Autodesk Inventor part; units mm, degrees
(part 2 of 6)
  line L1007 (12.5, 39) -> (11.5, 39)
  line L1008 (11.5, 37.2) -> (11.5, 36.2)
  line L1009 (11.5, 36.2) -> (12.5, 36.2)
  line L1010 (12.5, 36.2) -> (12.5, 37.2)
  line L1011 (12.5, 37.2) -> (11.5, 37.2)
  line L1012 (4.542, 13.47) -> (5.542, 13.47)
  line L1013 (5.542, 13.47) -> (5.542, 14.47)
  line L1014 (5.542, 14.47) -> (4.542, 14.47)
  line L1015 (4.542, 14.47) -> (4.542, 13.47)
  line L1016 (6.142, 13.47) -> (7.142, 13.47)
  line L1017 (7.142, 13.47) -> (7.142, 14.47)
  line L1018 (7.142, 14.47) -> (6.142, 14.47)
  line L1019 (6.142, 14.47) -> (6.142, 13.47)
  line L1020 (7.142, 20.058) -> (6.142, 20.058)
  line L1021 (6.142, 20.058) -> (6.142, 19.058)
  line L1022 (6.142, 19.058) -> (7.142, 19.058)
  line L1023 (7.142, 19.058) -> (7.142, 20.058)
  line L1024 (5.542, 20.058) -> (4.542, 20.058)
  line L1025 (4.542, 20.058) -> (4.542, 19.058)
  line L1026 (4.542, 19.058) -> (5.542, 19.058)
  line L1027 (5.542, 19.058) -> (5.542, 20.058)
  line L1028 (28.0642, 20.3777) -> (28.7713, 19.6706)
  line L1029 (28.7713, 19.6706) -> (29.4784, 20.3777)
  line L1030 (29.4784, 20.3777) -> (28.7713, 21.0848)
  line L1031 (28.7713, 21.0848) -> (28.0642, 20.3777)
  line L1032 (29.1956, 19.2463) -> (29.9027, 18.5392)
  line L1033 (29.9027, 18.5392) -> (30.6098, 19.2463)
  line L1034 (30.6098, 19.2463) -> (29.9027, 19.9534)
  line L1035 (29.9027, 19.9534) -> (29.1956, 19.2463)
  line L1036 (20.985, 6.977) -> (19.985, 6.977)
  line L1037 (19.985, 6.977) -> (19.985, 5.977)
  line L1038 (19.985, 5.977) -> (20.985, 5.977)
  line L1039 (20.985, 5.977) -> (20.985, 6.977)
  line L1040 (19.385, 6.977) -> (18.385, 6.977)
  line L1041 (18.385, 6.977) -> (18.385, 5.977)
  line L1042 (18.385, 5.977) -> (19.385, 5.977)
  line L1043 (19.385, 5.977) -> (19.385, 6.977)
  line L1044 (17.981, 1.829) -> (18.981, 1.829)
  line L1045 (18.981, 1.829) -> (18.981, 2.829)
  line L1046 (18.981, 2.829) -> (17.981, 2.829)
  line L1047 (17.981, 2.829) -> (17.981, 1.829)
  line L1048 (19.881, 1.829) -> (20.881, 1.829)
  line L1049 (20.881, 1.829) -> (20.881, 2.829)
  line L1050 (20.881, 2.829) -> (19.881, 2.829)
  line L1051 (19.881, 2.829) -> (19.881, 1.829)
  line L1052 (18.931, 4.029) -> (19.931, 4.029)
  line L1053 (19.931, 4.029) -> (19.931, 5.029)
  line L1054 (19.931, 5.029) -> (18.931, 5.029)
  line L1055 (18.931, 5.029) -> (18.931, 4.029)
  circle A10 centre (7.874, 6.096) radius 0.5
  circle A11 centre (7.874, 43.053) radius 0.5
  circle A12 centre (27.94, 43.053) radius 0.5
  circle A13 centre (7.874, 6.096) radius 0.5
  circle A14 centre (7.874, 43.053) radius 0.5
  circle A15 centre (27.94, 43.053) radius 0.5
  circle A16 centre (3.302, 41.148) radius 2.667
  circle A17 centre (3.302, 41.148) radius 1.908
  circle A18 centre (3.302, 41.148) radius 1.908
  circle A19 centre (3.302, 41.148) radius 2.667
  circle A20 centre (32.258, 41.148) radius 2.667
  circle A21 centre (32.258, 41.148) radius 1.908
  circle A22 centre (32.258, 41.148) radius 1.908
  circle A23 centre (32.258, 41.148) radius 2.667
  line L1056 (33.0454, 18.9463) -> (33.0454, 19.6617)
  line L1057 (33.0454, 19.6617) -> (33.5513, 20.1676)
  line L1058 (33.5513, 20.1676) -> (34.2667, 20.1676)
  line L1059 (34.2667, 20.1676) -> (34.7726, 19.6617)
  line L1060 (34.7726, 19.6617) -> (34.7726, 18.9463)
  line L1061 (34.7726, 18.9463) -> (34.2667, 18.4404)
  line L1062 (34.2667, 18.4404) -> (33.5513, 18.4404)
  line L1063 (33.5513, 18.4404) -> (33.0454, 18.9463)
  circle A24 centre (33.909, 19.304) radius 0.8636
  circle A25 centre (33.909, 19.304) radius 0.8636
  line L1064 (33.0454, 18.9463) -> (33.0454, 19.6617)
  line L1065 (33.0454, 19.6617) -> (33.5513, 20.1676)
  line L1066 (33.5513, 20.1676) -> (34.2667, 20.1676)
  line L1067 (34.2667, 20.1676) -> (34.7726, 19.6617)
  line L1068 (34.7726, 19.6617) -> (34.7726, 18.9463)
  line L1069 (34.7726, 18.9463) -> (34.2667, 18.4404)
  line L1070 (34.2667, 18.4404) -> (33.5513, 18.4404)
  line L1071 (33.5513, 18.4404) -> (33.0454, 18.9463)
  line L1072 (33.0454, 16.4063) -> (33.0454, 17.1217)
  line L1073 (33.0454, 17.1217) -> (33.5513, 17.6276)
  line L1074 (33.5513, 17.6276) -> (34.2667, 17.6276)
  line L1075 (34.2667, 17.6276) -> (34.7726, 17.1217)
  line L1076 (34.7726, 17.1217) -> (34.7726, 16.4063)
  line L1077 (34.7726, 16.4063) -> (34.2667, 15.9004)
  line L1078 (34.2667, 15.9004) -> (33.5513, 15.9004)
  line L1079 (33.5513, 15.9004) -> (33.0454, 16.4063)
  circle A26 centre (33.909, 16.764) radius 0.8636
  circle A27 centre (33.909, 16.764) radius 0.8636
  line L1080 (33.0454, 16.4063) -> (33.0454, 17.1217)
  line L1081 (33.0454, 17.1217) -> (33.5513, 17.6276)
  line L1082 (33.5513, 17.6276) -> (34.2667, 17.6276)
  line L1083 (34.2667, 17.6276) -> (34.7726, 17.1217)
  line L1084 (34.7726, 17.1217) -> (34.7726, 16.4063)
  line L1085 (34.7726, 16.4063) -> (34.2667, 15.9004)
  line L1086 (34.2667, 15.9004) -> (33.5513, 15.9004)
  line L1087 (33.5513, 15.9004) -> (33.0454, 16.4063)
  line L1088 (33.0454, 13.8663) -> (33.0454, 14.5817)
  line L1089 (33.0454, 14.5817) -> (33.5513, 15.0876)
  line L1090 (33.5513, 15.0876) -> (34.2667, 15.0876)
  line L1091 (34.2667, 15.0876) -> (34.7726, 14.5817)
  line L1092 (34.7726, 14.5817) -> (34.7726, 13.8663)
  line L1093 (34.7726, 13.8663) -> (34.2667, 13.3604)
  line L1094 (34.2667, 13.3604) -> (33.5513, 13.3604)
  line L1095 (33.5513, 13.3604) -> (33.0454, 13.8663)
  circle A28 centre (33.909, 14.224) radius 0.8636
  circle A29 centre (33.909, 14.224) radius 0.8636
  line L1096 (33.0454, 13.8663) -> (33.0454, 14.5817)
  line L1097 (33.0454, 14.5817) -> (33.5513, 15.0876)
  line L1098 (33.5513, 15.0876) -> (34.2667, 15.0876)
  line L1099 (34.2667, 15.0876) -> (34.7726, 14.5817)
  line L1100 (34.7726, 14.5817) -> (34.7726, 13.8663)
  line L1101 (34.7726, 13.8663) -> (34.2667, 13.3604)
  line L1102 (34.2667, 13.3604) -> (33.5513, 13.3604)
  line L1103 (33.5513, 13.3604) -> (33.0454, 13.8663)
  line L1104 (33.0454, 11.3263) -> (33.0454, 12.0417)
  line L1105 (33.0454, 12.0417) -> (33.5513, 12.5476)
  line L1106 (33.5513, 12.5476) -> (34.2667, 12.5476)
  line L1107 (34.2667, 12.5476) -> (34.7726, 12.0417)
  line L1108 (34.7726, 12.0417) -> (34.7726, 11.3263)
  line L1109 (34.7726, 11.3263) -> (34.2667, 10.8204)
  line L1110 (34.2667, 10.8204) -> (33.5513, 10.8204)
  line L1111 (33.5513, 10.8204) -> (33.0454, 11.3263)
  circle A30 centre (33.909, 11.684) radius 0.8636
  circle A31 centre (33.909, 11.684) radius 0.8636
  line L1112 (33.0454, 11.3263) -> (33.0454, 12.0417)
  line L1113 (33.0454, 12.0417) -> (33.5513, 12.5476)
  line L1114 (33.5513, 12.5476) -> (34.2667, 12.5476)
  line L1115 (34.2667, 12.5476) -> (34.7726, 12.0417)
  line L1116 (34.7726, 12.0417) -> (34.7726, 11.3263)
  line L1117 (34.7726, 11.3263) -> (34.2667, 10.8204)
  line L1118 (34.2667, 10.8204) -> (33.5513, 10.8204)
  line L1119 (33.5513, 10.8204) -> (33.0454, 11.3263)
  line L1120 (33.0454, 8.7863) -> (33.0454, 9.5017)
  line L1121 (33.0454, 9.5017) -> (33.5513, 10.0076)
  line L1122 (33.5513, 10.0076) -> (34.2667, 10.0076)
  line L1123 (34.2667, 10.0076) -> (34.7726, 9.5017)
  line L1124 (34.7726, 9.5017) -> (34.7726, 8.7863)
  line L1125 (34.7726, 8.7863) -> (34.2667, 8.2804)
  line L1126 (34.2667, 8.2804) -> (33.5513, 8.2804)
  line L1127 (33.5513, 8.2804) -> (33.0454, 8.7863)
  circle A32 centre (33.909, 9.144) radius 0.8636
  circle A33 centre (33.909, 9.144) radius 0.8636
  line L1128 (33.0454, 8.7863) -> (33.0454, 9.5017)
  line L1129 (33.0454, 9.5017) -> (33.5513, 10.0076)
  line L1130 (33.5513, 10.0076) -> (34.2667, 10.0076)
  line L1131 (34.2667, 10.0076) -> (34.7726, 9.5017)
  line L1132 (34.7726, 9.5017) -> (34.7726, 8.7863)
  line L1133 (34.7726, 8.7863) -> (34.2667, 8.2804)
  line L1134 (34.2667, 8.2804) -> (33.5513, 8.2804)
  line L1135 (33.5513, 8.2804) -> (33.0454, 8.7863)
  line L1136 (33.0454, 6.2463) -> (33.0454, 6.9617)
  line L1137 (33.0454, 6.9617) -> (33.5513, 7.4676)
  line L1138 (33.5513, 7.4676) -> (34.2667, 7.4676)
  line L1139 (34.2667, 7.4676) -> (34.7726, 6.9617)
  line L1140 (34.7726, 6.9617) -> (34.7726, 6.2463)
  line L1141 (34.7726, 6.2463) -> (34.2667, 5.7404)
  line L1142 (34.2667, 5.7404) -> (33.5513, 5.7404)
  line L1143 (33.5513, 5.7404) -> (33.0454, 6.2463)
  circle A34 centre (33.909, 6.604) radius 0.8636
  circle A35 centre (33.909, 6.604) radius 0.8636
  line L1144 (33.0454, 6.2463) -> (33.0454, 6.9617)
  line L1145 (33.0454, 6.9617) -> (33.5513, 7.4676)
  line L1146 (33.5513, 7.4676) -> (34.2667, 7.4676)
  line L1147 (34.2667, 7.4676) -> (34.7726, 6.9617)
  line L1148 (34.7726, 6.9617) -> (34.7726, 6.2463)
  line L1149 (34.7726, 6.2463) -> (34.2667, 5.7404)
  line L1150 (34.2667, 5.7404) -> (33.5513, 5.7404)
  line L1151 (33.5513, 5.7404) -> (33.0454, 6.2463)
  line L1152 (33.0454, 3.7063) -> (33.0454, 4.4217)
  line L1153 (33.0454, 4.4217) -> (33.5513, 4.9276)
  line L1154 (33.5513, 4.9276) -> (34.2667, 4.9276)
  line L1155 (34.2667, 4.9276) -> (34.7726, 4.4217)
  line L1156 (34.7726, 4.4217) -> (34.7726, 3.7063)
  line L1157 (34.7726, 3.7063) -> (34.2667, 3.2004)
  line L1158 (34.2667, 3.2004) -> (33.5513, 3.2004)
  line L1159 (33.5513, 3.2004) -> (33.0454, 3.7063)
  circle A36 centre (33.909, 4.064) radius 0.8636
  circle A37 centre (33.909, 4.064) radius 0.8636
  line L1160 (33.0454, 3.7063) -> (33.0454, 4.4217)
  line L1161 (33.0454, 4.4217) -> (33.5513, 4.9276)
  line L1162 (33.5513, 4.9276) -> (34.2667, 4.9276)
  line L1163 (34.2667, 4.9276) -> (34.7726, 4.4217)
  line L1164 (34.7726, 4.4217) -> (34.7726, 3.7063)
  line L1165 (34.7726, 3.7063) -> (34.2667, 3.2004)
  line L1166 (34.2667, 3.2004) -> (33.5513, 3.2004)
  line L1167 (33.5513, 3.2004) -> (33.0454, 3.7063)
  line L1168 (33.0454, 1.1663) -> (33.0454, 1.8817)
  line L1169 (33.0454, 1.8817) -> (33.5513, 2.3876)
  line L1170 (33.5513, 2.3876) -> (34.2667, 2.3876)
  line L1171 (34.2667, 2.3876) -> (34.7726, 1.8817)
  line L1172 (34.7726, 1.8817) -> (34.7726, 1.1663)
  line L1173 (34.7726, 1.1663) -> (34.2667, 0.6604)
  line L1174 (34.2667, 0.6604) -> (33.5513, 0.6604)
  line L1175 (33.5513, 0.6604) -> (33.0454, 1.1663)
  circle A38 centre (33.909, 1.524) radius 0.8636
  circle A39 centre (33.909, 1.524) radius 0.8636
  line L1176 (33.0454, 1.1663) -> (33.0454, 1.8817)
  line L1177 (33.0454, 1.8817) -> (33.5513, 2.3876)
  line L1178 (33.5513, 2.3876) -> (34.2667, 2.3876)
  line L1179 (34.2667, 2.3876) -> (34.7726, 1.8817)
  line L1180 (34.7726, 1.8817) -> (34.7726, 1.1663)
  line L1181 (34.7726, 1.1663) -> (34.2667, 0.6604)
  line L1182 (34.2667, 0.6604) -> (33.5513, 0.6604)
  line L1183 (33.5513, 0.6604) -> (33.0454, 1.1663)
  line L1184 (0.7874, 18.9463) -> (0.7874, 19.6617)
  line L1185 (0.7874, 19.6617) -> (1.2933, 20.1676)
  line L1186 (1.2933, 20.1676) -> (2.0087, 20.1676)
  line L1187 (2.0087, 20.1676) -> (2.5146, 19.6617)
  line L1188 (2.5146, 19.6617) -> (2.5146, 18.9463)
  line L1189 (2.5146, 18.9463) -> (2.0087, 18.4404)
  line L1190 (2.0087, 18.4404) -> (1.2933, 18.4404)
  line L1191 (1.2933, 18.4404) -> (0.7874, 18.9463)
  circle A40 centre (1.651, 19.304) radius 0.8636
  circle A41 centre (1.651, 19.304) radius 0.8636
  line L1192 (0.7874, 18.9463) -> (0.7874, 19.6617)
  line L1193 (0.7874, 19.6617) -> (1.2933, 20.1676)
  line L1194 (1.2933, 20.1676) -> (2.0087, 20.1676)
  line L1195 (2.0087, 20.1676) -> (2.5146, 19.6617)
  line L1196 (2.5146, 19.6617) -> (2.5146, 18.9463)
  line L1197 (2.5146, 18.9463) -> (2.0087, 18.4404)
  line L1198 (2.0087, 18.4404) -> (1.2933, 18.4404)
  line L1199 (1.2933, 18.4404) -> (0.7874, 18.9463)
  line L1200 (0.7874, 16.4063) -> (0.7874, 17.1217)
  line L1201 (0.7874, 17.1217) -> (1.2933, 17.6276)
  line L1202 (1.2933, 17.6276) -> (2.0087, 17.6276)
  line L1203 (2.0087, 17.6276) -> (2.5146, 17.1217)
  line L1204 (2.5146, 17.1217) -> (2.5146, 16.4063)
  line L1205 (2.5146, 16.4063) -> (2.0087, 15.9004)
  line L1206 (2.0087, 15.9004) -> (1.2933, 15.9004)
  line L1207 (1.2933, 15.9004) -> (0.7874, 16.4063)
  circle A42 centre (1.651, 16.764) radius 0.8636
  circle A43 centre (1.651, 16.764) radius 0.8636
  line L1208 (0.7874, 16.4063) -> (0.7874, 17.1217)
  line L1209 (0.7874, 17.1217) -> (1.2933, 17.6276)
  line L1210 (1.2933, 17.6276) -> (2.0087, 17.6276)
  line L1211 (2.0087, 17.6276) -> (2.5146, 17.1217)
  line L1212 (2.5146, 17.1217) -> (2.5146, 16.4063)
  line L1213 (2.5146, 16.4063) -> (2.0087, 15.9004)
  line L1214 (2.0087, 15.9004) -> (1.2933, 15.9004)
  line L1215 (1.2933, 15.9004) -> (0.7874, 16.4063)
  line L1216 (0.7874, 13.8663) -> (0.7874, 14.5817)
  line L1217 (0.7874, 14.5817) -> (1.2933, 15.0876)
  line L1218 (1.2933, 15.0876) -> (2.0087, 15.0876)
  line L1219 (2.0087, 15.0876) -> (2.5146, 14.5817)
  line L1220 (2.5146, 14.5817) -> (2.5146, 13.8663)
  line L1221 (2.5146, 13.8663) -> (2.0087, 13.3604)
  line L1222 (2.0087, 13.3604) -> (1.2933, 13.3604)
  line L1223 (1.2933, 13.3604) -> (0.7874, 13.8663)
  circle A44 centre (1.651, 14.224) radius 0.8636
  circle A45 centre (1.651, 14.224) radius 0.8636
  line L1224 (0.7874, 13.8663) -> (0.7874, 14.5817)
  line L1225 (0.7874, 14.5817) -> (1.2933, 15.0876)
  line L1226 (1.2933, 15.0876) -> (2.0087, 15.0876)
  line L1227 (2.0087, 15.0876) -> (2.5146, 14.5817)
  line L1228 (2.5146, 14.5817) -> (2.5146, 13.8663)
  line L1229 (2.5146, 13.8663) -> (2.0087, 13.3604)
  line L1230 (2.0087, 13.3604) -> (1.2933, 13.3604)
  line L1231 (1.2933, 13.3604) -> (0.7874, 13.8663)
  line L1232 (0.7874, 11.3263) -> (0.7874, 12.0417)
  line L1233 (0.7874, 12.0417) -> (1.2933, 12.5476)
  line L1234 (1.2933, 12.5476) -> (2.0087, 12.5476)
  line L1235 (2.0087, 12.5476) -> (2.5146, 12.0417)
  line L1236 (2.5146, 12.0417) -> (2.5146, 11.3263)
  line L1237 (2.5146, 11.3263) -> (2.0087, 10.8204)
  line L1238 (2.0087, 10.8204) -> (1.2933, 10.8204)
  line L1239 (1.2933, 10.8204) -> (0.7874, 11.3263)
  circle A46 centre (1.651, 11.684) radius 0.8636
  circle A47 centre (1.651, 11.684) radius 0.8636
  line L1240 (0.7874, 11.3263) -> (0.7874, 12.0417)
  line L1241 (0.7874, 12.0417) -> (1.2933, 12.5476)
  line L1242 (1.2933, 12.5476) -> (2.0087, 12.5476)
  line L1243 (2.0087, 12.5476) -> (2.5146, 12.0417)
  line L1244 (2.5146, 12.0417) -> (2.5146, 11.3263)
  line L1245 (2.5146, 11.3263) -> (2.0087, 10.8204)
  line L1246 (2.0087, 10.8204) -> (1.2933, 10.8204)
  line L1247 (1.2933, 10.8204) -> (0.7874, 11.3263)
  line L1248 (0.7874, 8.7863) -> (0.7874, 9.5017)
  line L1249 (0.7874, 9.5017) -> (1.2933, 10.0076)
  line L1250 (1.2933, 10.0076) -> (2.0087, 10.0076)
  line L1251 (2.0087, 10.0076) -> (2.5146, 9.5017)
  line L1252 (2.5146, 9.5017) -> (2.5146, 8.7863)
  line L1253 (2.5146, 8.7863) -> (2.0087, 8.2804)
  line L1254 (2.0087, 8.2804) -> (1.2933, 8.2804)
  line L1255 (1.2933, 8.2804) -> (0.7874, 8.7863)
  circle A48 centre (1.651, 9.144) radius 0.8636
  circle A49 centre (1.651, 9.144) radius 0.8636
  line L1256 (0.7874, 8.7863) -> (0.7874, 9.5017)
  line L1257 (0.7874, 9.5017) -> (1.2933, 10.0076)
  line L1258 (1.2933, 10.0076) -> (2.0087, 10.0076)
  line L1259 (2.0087, 10.0076) -> (2.5146, 9.5017)
  line L1260 (2.5146, 9.5017) -> (2.5146, 8.7863)
  line L1261 (2.5146, 8.7863) -> (2.0087, 8.2804)
  line L1262 (2.0087, 8.2804) -> (1.2933, 8.2804)
  line L1263 (1.2933, 8.2804) -> (0.7874, 8.7863)
  line L1264 (0.7874, 6.2463) -> (0.7874, 6.9617)
  line L1265 (0.7874, 6.9617) -> (1.2933, 7.4676)
  line L1266 (1.2933, 7.4676) -> (2.0087, 7.4676)
  line L1267 (2.0087, 7.4676) -> (2.5146, 6.9617)
  line L1268 (2.5146, 6.9617) -> (2.5146, 6.2463)
  line L1269 (2.5146, 6.2463) -> (2.0087, 5.7404)
  line L1270 (2.0087, 5.7404) -> (1.2933, 5.7404)
  line L1271 (1.2933, 5.7404) -> (0.7874, 6.2463)
  circle A50 centre (1.651, 6.604) radius 0.8636
  circle A51 centre (1.651, 6.604) radius 0.8636
  line L1272 (0.7874, 6.2463) -> (0.7874, 6.9617)
  line L1273 (0.7874, 6.9617) -> (1.2933, 7.4676)
  line L1274 (1.2933, 7.4676) -> (2.0087, 7.4676)
  line L1275 (2.0087, 7.4676) -> (2.5146, 6.9617)
  line L1276 (2.5146, 6.9617) -> (2.5146, 6.2463)
  line L1277 (2.5146, 6.2463) -> (2.0087, 5.7404)
  line L1278 (2.0087, 5.7404) -> (1.2933, 5.7404)
  line L1279 (1.2933, 5.7404) -> (0.7874, 6.2463)
  line L1280 (0.7874, 3.7063) -> (0.7874, 4.4217)
  line L1281 (0.7874, 4.4217) -> (1.2933, 4.9276)
  line L1282 (1.2933, 4.9276) -> (2.0087, 4.9276)
  line L1283 (2.0087, 4.9276) -> (2.5146, 4.4217)
  line L1284 (2.5146, 4.4217) -> (2.5146, 3.7063)
  line L1285 (2.5146, 3.7063) -> (2.0087, 3.2004)
  line L1286 (2.0087, 3.2004) -> (1.2933, 3.2004)
  line L1287 (1.2933, 3.2004) -> (0.7874, 3.7063)
  circle A52 centre (1.651, 4.064) radius 0.8636
  circle A53 centre (1.651, 4.064) radius 0.8636
  line L1288 (0.7874, 3.7063) -> (0.7874, 4.4217)
  line L1289 (0.7874, 4.4217) -> (1.2933, 4.9276)
  line L1290 (1.2933, 4.9276) -> (2.0087, 4.9276)
  line L1291 (2.0087, 4.9276) -> (2.5146, 4.4217)
  line L1292 (2.5146, 4.4217) -> (2.5146, 3.7063)
  line L1293 (2.5146, 3.7063) -> (2.0087, 3.2004)
  line L1294 (2.0087, 3.2004) -> (1.2933, 3.2004)
  line L1295 (1.2933, 3.2004) -> (0.7874, 3.7063)
  line L1296 (0.7874, 1.1663) -> (0.7874, 1.8817)
  line L1297 (0.7874, 1.8817) -> (1.2933, 2.3876)
  line L1298 (1.2933, 2.3876) -> (2.0087, 2.3876)
  line L1299 (2.0087, 2.3876) -> (2.5146, 1.8817)
  line L1300 (2.5146, 1.8817) -> (2.5146, 1.1663)
  line L1301 (2.5146, 1.1663) -> (2.0087, 0.6604)
  line L1302 (2.0087, 0.6604) -> (1.2933, 0.6604)
  line L1303 (1.2933, 0.6604) -> (0.7874, 1.1663)
  circle A54 centre (1.651, 1.524) radius 0.8636
  circle A55 centre (1.651, 1.524) radius 0.8636
  line L1304 (0.7874, 1.1663) -> (0.7874, 1.8817)
  line L1305 (0.7874, 1.8817) -> (1.2933, 2.3876)
  line L1306 (1.2933, 2.3876) -> (2.0087, 2.3876)
  line L1307 (2.0087, 2.3876) -> (2.5146, 1.8817)
  line L1308 (2.5146, 1.8817) -> (2.5146, 1.1663)
  line L1309 (2.5146, 1.1663) -> (2.0087, 0.6604)
  line L1310 (2.0087, 0.6604) -> (1.2933, 0.6604)
  line L1311 (1.2933, 0.6604) -> (0.7874, 1.1663)
  line L1312 (29.2354, 16.4063) -> (29.2354, 17.1217)
  line L1313 (29.2354, 17.1217) -> (29.7413, 17.6276)
  line L1314 (29.7413, 17.6276) -> (30.4567, 17.6276)
  line L1315 (30.4567, 17.6276) -> (30.9626, 17.1217)
  line L1316 (30.9626, 17.1217) -> (30.9626, 16.4063)
  line L1317 (30.9626, 16.4063) -> (30.4567, 15.9004)
  line L1318 (30.4567, 15.9004) -> (29.7413, 15.9004)
  line L1319 (29.7413, 15.9004) -> (29.2354, 16.4063)
  circle A56 centre (30.099, 16.764) radius 0.8636
  circle A57 centre (30.099, 16.764) radius 0.8636
  line L1320 (29.2354, 16.4063) -> (29.2354, 17.1217)
  line L1321 (29.2354, 17.1217) -> (29.7413, 17.6276)
  line L1322 (29.7413, 17.6276) -> (30.4567, 17.6276)
  line L1323 (30.4567, 17.6276) -> (30.9626, 17.1217)
  line L1324 (30.9626, 17.1217) -> (30.9626, 16.4063)
  line L1325 (30.9626, 16.4063) -> (30.4567, 15.9004)
  line L1326 (30.4567, 15.9004) -> (29.7413, 15.9004)
  line L1327 (29.7413, 15.9004) -> (29.2354, 16.4063)
  line L1328 (29.2354, 13.8663) -> (29.2354, 14.5817)
  line L1329 (29.2354, 14.5817) -> (29.7413, 15.0876)
  line L1330 (29.7413, 15.0876) -> (30.4567, 15.0876)
  line L1331 (30.4567, 15.0876) -> (30.9626, 14.5817)
  line L1332 (30.9626, 14.5817) -> (30.9626, 13.8663)
  line L1333 (30.9626, 13.8663) -> (30.4567, 13.3604)
  line L1334 (30.4567, 13.3604) -> (29.7413, 13.3604)
  line L1335 (29.7413, 13.3604) -> (29.2354, 13.8663)
  circle A58 centre (30.099, 14.224) radius 0.8636
  circle A59 centre (30.099, 14.224) radius 0.8636
  line L1336 (29.2354, 13.8663) -> (29.2354, 14.5817)
  line L1337 (29.2354, 14.5817) -> (29.7413, 15.0876)
  line L1338 (29.7413, 15.0876) -> (30.4567, 15.0876)
  line L1339 (30.4567, 15.0876) -> (30.9626, 14.5817)
  line L1340 (30.9626, 14.5817) -> (30.9626, 13.8663)
  line L1341 (30.9626, 13.8663) -> (30.4567, 13.3604)
  line L1342 (30.4567, 13.3604) -> (29.7413, 13.3604)
  line L1343 (29.7413, 13.3604) -> (29.2354, 13.8663)
  line L1344 (29.2354, 11.3263) -> (29.2354, 12.0417)
  line L1345 (29.2354, 12.0417) -> (29.7413, 12.5476)
  line L1346 (29.7413, 12.5476) -> (30.4567, 12.5476)
  line L1347 (30.4567, 12.5476) -> (30.9626, 12.0417)
  line L1348 (30.9626, 12.0417) -> (30.9626, 11.3263)
  line L1349 (30.9626, 11.3263) -> (30.4567, 10.8204)
  line L1350 (30.4567, 10.8204) -> (29.7413, 10.8204)
  line L1351 (29.7413, 10.8204) -> (29.2354, 11.3263)
  circle A60 centre (30.099, 11.684) radius 0.8636
  circle A61 centre (30.099, 11.684) radius 0.8636
  line L1352 (29.2354, 11.3263) -> (29.2354, 12.0417)
  line L1353 (29.2354, 12.0417) -> (29.7413, 12.5476)
  line L1354 (29.7413, 12.5476) -> (30.4567, 12.5476)
  line L1355 (30.4567, 12.5476) -> (30.9626, 12.0417)
  line L1356 (30.9626, 12.0417) -> (30.9626, 11.3263)
  line L1357 (30.9626, 11.3263) -> (30.4567, 10.8204)
  line L1358 (30.4567, 10.8204) -> (29.7413, 10.8204)
  line L1359 (29.7413, 10.8204) -> (29.2354, 11.3263)
  line L1360 (29.2354, 8.7863) -> (29.2354, 9.5017)
  line L1361 (29.2354, 9.5017) -> (29.7413, 10.0076)
  line L1362 (29.7413, 10.0076) -> (30.4567, 10.0076)
  line L1363 (30.4567, 10.0076) -> (30.9626, 9.5017)
  line L1364 (30.9626, 9.5017) -> (30.9626, 8.7863)
  line L1365 (30.9626, 8.7863) -> (30.4567, 8.2804)
  line L1366 (30.4567, 8.2804) -> (29.7413, 8.2804)
  line L1367 (29.7413, 8.2804) -> (29.2354, 8.7863)
  circle A62 centre (30.099, 9.144) radius 0.8636
  circle A63 centre (30.099, 9.144) radius 0.8636
  line L1368 (29.2354, 8.7863) -> (29.2354, 9.5017)
  line L1369 (29.2354, 9.5017) -> (29.7413, 10.0076)
  line L1370 (29.7413, 10.0076) -> (30.4567, 10.0076)
  line L1371 (30.4567, 10.0076) -> (30.9626, 9.5017)
  line L1372 (30.9626, 9.5017) -> (30.9626, 8.7863)
  line L1373 (30.9626, 8.7863) -> (30.4567, 8.2804)
  line L1374 (30.4567, 8.2804) -> (29.7413, 8.2804)
  line L1375 (29.7413, 8.2804) -> (29.2354, 8.7863)
  line L1376 (29.2354, 6.2463) -> (29.2354, 6.9617)
  line L1377 (29.2354, 6.9617) -> (29.7413, 7.4676)
  line L1378 (29.7413, 7.4676) -> (30.4567, 7.4676)
  line L1379 (30.4567, 7.4676) -> (30.9626, 6.9617)
  line L1380 (30.9626, 6.9617) -> (30.9626, 6.2463)
  line L1381 (30.9626, 6.2463) -> (30.4567, 5.7404)
  line L1382 (30.4567, 5.7404) -> (29.7413, 5.7404)
  line L1383 (29.7413, 5.7404) -> (29.2354, 6.2463)
  circle A64 centre (30.099, 6.604) radius 0.8636
  circle A65 centre (30.099, 6.604) radius 0.8636
  line L1384 (29.2354, 6.2463) -> (29.2354, 6.9617)
  line L1385 (29.2354, 6.9617) -> (29.7413, 7.4676)
  line L1386 (29.7413, 7.4676) -> (30.4567, 7.4676)
  line L1387 (30.4567, 7.4676) -> (30.9626, 6.9617)
  line L1388 (30.9626, 6.9617) -> (30.9626, 6.2463)
  line L1389 (30.9626, 6.2463) -> (30.4567, 5.7404)
  line L1390 (30.4567, 5.7404) -> (29.7413, 5.7404)
  line L1391 (29.7413, 5.7404) -> (29.2354, 6.2463)
  line L1392 (4.453, 11.714) -> (4.453, 10.714)
  line L1393 (4.453, 10.714) -> (5.453, 10.714)
  line L1394 (5.453, 10.714) -> (5.453, 11.714)
  line L1395 (5.453, 11.714) -> (4.453, 11.714)
  line L1396 (4.453, 10.114) -> (4.453, 9.114)
  line L1397 (4.453, 9.114) -> (5.453, 9.114)
  line L1398 (5.453, 9.114) -> (5.453, 10.114)
  line L1399 (5.453, 10.114) -> (4.453, 10.114)
  line L1400 (24.287, 6.977) -> (23.287, 6.977)
  line L1401 (23.287, 6.977) -> (23.287, 5.977)
  line L1402 (23.287, 5.977) -> (24.287, 5.977)
  line L1403 (24.287, 5.977) -> (24.287, 6.977)
  line L1404 (22.687, 6.977) -> (21.687, 6.977)
  line L1405 (21.687, 6.977) -> (21.687, 5.977)
  line L1406 (21.687, 5.977) -> (22.687, 5.977)
  line L1407 (22.687, 5.977) -> (22.687, 6.977)
  line L1408 (2.74, 31.099) -> (3.74, 31.099)
  line L1409 (3.74, 31.099) -> (3.74, 32.099)
  line L1410 (3.74, 32.099) -> (2.74, 32.099)
  line L1411 (2.74, 32.099) -> (2.74, 31.099)
  line L1412 (2.74, 28.099) -> (3.74, 28.099)
  line L1413 (3.74, 28.099) -> (3.74, 29.099)
  line L1414 (3.74, 29.099) -> (2.74, 29.099)
  line L1415 (2.74, 29.099) -> (2.74, 28.099)
  line L1416 (1.34, 28.099) -> (2.34, 28.099)
  line L1417 (2.34, 28.099) -> (2.34, 29.099)
  line L1418 (2.34, 29.099) -> (1.34, 29.099)
  line L1419 (1.34, 29.099) -> (1.34, 28.099)
  line L1420 (1.34, 31.099) -> (2.34, 31.099)
  line L1421 (2.34, 31.099) -> (2.34, 32.099)
  line L1422 (2.34, 32.099) -> (1.34, 32.099)
  line L1423 (1.34, 32.099) -> (1.34, 31.099)
  line L1424 (34.8585, 34.5556) -> (34.1514, 35.2627)
  line L1425 (34.1514, 35.2627) -> (33.4443, 34.5556)
  line L1426 (33.4443, 34.5556) -> (34.1514, 33.8485)
  line L1427 (34.1514, 33.8485) -> (34.8585, 34.5556)
  line L1428 (32.5957, 36.8184) -> (31.8886, 37.5255)
  line L1429 (31.8886, 37.5255) -> (31.1815, 36.8184)
  line L1430 (31.1815, 36.8184) -> (31.8886, 36.1113)
  line L1431 (31.8886, 36.1113) -> (32.5957, 36.8184)
  line L1432 (3.6714, 37.5255) -> (2.9643, 36.8184)
  line L1433 (2.9643, 36.8184) -> (3.6714, 36.1113)
  line L1434 (3.6714, 36.1113) -> (4.3785, 36.8184)
  line L1435 (4.3785, 36.8184) -> (3.6714, 37.5255)
  line L1436 (1.4086, 35.2627) -> (0.7015, 34.5556)
  line L1437 (0.7015, 34.5556) -> (1.4086, 33.8485)
  line L1438 (1.4086, 33.8485) -> (2.1157, 34.5556)
  line L1439 (2.1157, 34.5556) -> (1.4086, 35.2627)
  circle A66 centre (7.78, 36.068) radius 2.2225
  circle A67 centre (7.78, 36.068) radius 1.778
  circle A68 centre (7.78, 36.068) radius 1.778
  circle A69 centre (7.78, 36.068) radius 2.2225
  circle A70 centre (27.78, 36.068) radius 2.2225
  circle A71 centre (27.78, 36.068) radius 1.778
  circle A72 centre (27.78, 36.068) radius 1.778
  circle A73 centre (27.78, 36.068) radius 2.2225
  line L1440 (2.106, 23.519) -> (3.106, 23.519)
  line L1441 (3.106, 23.519) -> (3.106, 24.519)
  line L1442 (3.106, 24.519) -> (2.106, 24.519)
  line L1443 (2.106, 24.519) -> (2.106, 23.519)
  line L1444 (4.006, 23.519) -> (5.006, 23.519)
  line L1445 (5.006, 23.519) -> (5.006, 24.519)
  line L1446 (5.006, 24.519) -> (4.006, 24.519)
  line L1447 (4.006, 24.519) -> (4.006, 23.519)
  line L1448 (3.056, 25.619) -> (4.056, 25.619)
  line L1449 (4.056, 25.619) -> (4.056, 26.619)
  line L1450 (4.056, 26.619) -> (3.056, 26.619)
  line L1451 (3.056, 26.619) -> (3.056, 25.619)
  line L1452 (5.469, 25.519) -> (5.469, 24.519)
  line L1453 (5.469, 24.519) -> (6.469, 24.519)
  line L1454 (6.469, 24.519) -> (6.469, 25.519)
  line L1455 (6.469, 25.519) -> (5.469, 25.519)
  line L1456 (5.469, 26.369) -> (5.469, 25.369)
  line L1457 (5.469, 25.369) -> (6.469, 25.369)
  line L1458 (6.469, 25.369) -> (6.469, 26.369)
  line L1459 (6.469, 26.369) -> (5.469, 26.369)
  line L1460 (5.469, 24.669) -> (5.469, 23.669)
  line L1461 (5.469, 23.669) -> (6.469, 23.669)
  line L1462 (6.469, 23.669) -> (6.469, 24.669)
  line L1463 (6.469, 24.669) -> (5.469, 24.669)
  line L1464 (0.643, 25.519) -> (0.643, 24.519)
  line L1465 (0.643, 24.519) -> (1.643, 24.519)
  line L1466 (1.643, 24.519) -> (1.643, 25.519)
  line L1467 (1.643, 25.519) -> (0.643, 25.519)
  line L1468 (0.643, 26.369) -> (0.643, 25.369)
  line L1469 (0.643, 25.369) -> (1.643, 25.369)
  line L1470 (1.643, 25.369) -> (1.643, 26.369)
  line L1471 (1.643, 26.369) -> (0.643, 26.369)
  line L1472 (0.643, 24.669) -> (0.643, 23.669)
  line L1473 (0.643, 23.669) -> (1.643, 23.669)
  line L1474 (1.643, 23.669) -> (1.643, 24.669)
  line L1475 (1.643, 24.669) -> (0.643, 24.669)
  line L1476 (19.804, 30.599) -> (18.804, 30.599)
  line L1477 (18.804, 30.599) -> (18.804, 29.599)
  line L1478 (18.804, 29.599) -> (19.804, 29.599)
  line L1479 (19.804, 29.599) -> (19.804, 30.599)
  line L1480 (20.654, 30.599) -> (19.654, 30.599)
  line L1481 (19.654, 30.599) -> (19.654, 29.599)
  line L1482 (19.654, 29.599) -> (20.654, 29.599)
  line L1483 (20.654, 29.599) -> (20.654, 30.599)
  line L1484 (18.954, 30.599) -> (17.954, 30.599)
  line L1485 (17.954, 30.599) -> (17.954, 29.599)
  line L1486 (17.954, 29.599) -> (18.954, 29.599)
  line L1487 (18.954, 29.599) -> (18.954, 30.599)
  line L1488 (23.2, 32.7) -> (23.2, 31.7)
  line L1489 (23.2, 31.7) -> (24.2, 31.7)
  line L1490 (24.2, 31.7) -> (24.2, 32.7)
  line L1491 (24.2, 32.7) -> (23.2, 32.7)
  line L1492 (23.2, 33.55) -> (23.2, 32.55)
  line L1493 (23.2, 32.55) -> (24.2, 32.55)
  line L1494 (24.2, 32.55) -> (24.2, 33.55)
  line L1495 (24.2, 33.55) -> (23.2, 33.55)
  line L1496 (23.2, 31.85) -> (23.2, 30.85)
  line L1497 (23.2, 30.85) -> (24.2, 30.85)
  line L1498 (24.2, 30.85) -> (24.2, 31.85)
  line L1499 (24.2, 31.85) -> (23.2, 31.85)
  line L1500 (5.1385, 32.053) -> (5.1385, 31.053)
  line L1501 (5.1385, 31.053) -> (6.1385, 31.053)
  line L1502 (6.1385, 31.053) -> (6.1385, 32.053)
  line L1503 (6.1385, 32.053) -> (5.1385, 32.053)
  line L1504 (5.1385, 31.253) -> (5.1385, 30.253)
  line L1505 (5.1385, 30.253) -> (6.1385, 30.253)
  line L1506 (6.1385, 30.253) -> (6.1385, 31.253)
  line L1507 (6.1385, 31.253) -> (5.1385, 31.253)
  line L1508 (5.1385, 30.453) -> (5.1385, 29.453)
  line L1509 (5.1385, 29.453) -> (6.1385, 29.453)
  line L1510 (6.1385, 29.453) -> (6.1385, 30.453)
  line L1511 (6.1385, 30.453) -> (5.1385, 30.453)
  line L1512 (5.1385, 29.653) -> (5.1385, 28.653)
  line L1513 (5.1385, 28.653) -> (6.1385, 28.653)
  line L1514 (6.1385, 28.653) -> (6.1385, 29.653)
  line L1515 (6.1385, 29.653) -> (5.1385, 29.653)
  line L1516 (7.6885, 28.653) -> (7.6885, 29.653)
  line L1517 (7.6885, 29.653) -> (6.6885, 29.653)
  line L1518 (6.6885, 29.653) -> (6.6885, 28.653)
  line L1519 (6.6885, 28.653) -> (7.6885, 28.653)
  line L1520 (7.6885, 29.453) -> (7.6885, 30.453)
  line L1521 (7.6885, 30.453) -> (6.6885, 30.453)
  line L1522 (6.6885, 30.453) -> (6.6885, 29.453)
  line L1523 (6.6885, 29.453) -> (7.6885, 29.453)
  line L1524 (7.6885, 30.253) -> (7.6885, 31.253)
  line L1525 (7.6885, 31.253) -> (6.6885, 31.253)
  line L1526 (6.6885, 31.253) -> (6.6885, 30.253)
  line L1527 (6.6885, 30.253) -> (7.6885, 30.253)
  line L1528 (7.6885, 31.053) -> (7.6885, 32.053)
  line L1529 (7.6885, 32.053) -> (6.6885, 32.053)
  line L1530 (6.6885, 32.053) -> (6.6885, 31.053)
  line L1531 (6.6885, 31.053) -> (7.6885, 31.053)
  line L1532 (26.792, 24.941) -> (26.792, 23.941)
  line L1533 (26.792, 23.941) -> (27.792, 23.941)
  line L1534 (27.792, 23.941) -> (27.792, 24.941)
  line L1535 (27.792, 24.941) -> (26.792, 24.941)
  line L1536 (26.792, 24.141) -> (26.792, 23.141)
  line L1537 (26.792, 23.141) -> (27.792, 23.141)
  line L1538 (27.792, 23.141) -> (27.792, 24.141)
  line L1539 (27.792, 24.141) -> (26.792, 24.141)
  line L1540 (26.792, 23.341) -> (26.792, 22.341)
  line L1541 (26.792, 22.341) -> (27.792, 22.341)
  line L1542 (27.792, 22.341) -> (27.792, 23.341)
  line L1543 (27.792, 23.341) -> (26.792, 23.341)
  line L1544 (26.792, 22.541) -> (26.792, 21.541)
  line L1545 (26.792, 21.541) -> (27.792, 21.541)
  line L1546 (27.792, 21.541) -> (27.792, 22.541)
  line L1547 (27.792, 22.541) -> (26.792, 22.541)
  line L1548 (29.342, 21.541) -> (29.342, 22.541)
  line L1549 (29.342, 22.541) -> (28.342, 22.541)
  line L1550 (28.342, 22.541) -> (28.342, 21.541)
  line L1551 (28.342, 21.541) -> (29.342, 21.541)
  line L1552 (29.342, 22.341) -> (29.342, 23.341)
  line L1553 (29.342, 23.341) -> (28.342, 23.341)
  line L1554 (28.342, 23.341) -> (28.342, 22.341)
  line L1555 (28.342, 22.341) -> (29.342, 22.341)
  line L1556 (29.342, 23.141) -> (29.342, 24.141)
  line L1557 (29.342, 24.141) -> (28.342, 24.141)
  line L1558 (28.342, 24.141) -> (28.342, 23.141)
  line L1559 (28.342, 23.141) -> (29.342, 23.141)
  line L1560 (29.342, 23.941) -> (29.342, 24.941)
  line L1561 (29.342, 24.941) -> (28.342, 24.941)
  line L1562 (28.342, 24.941) -> (28.342, 23.941)
  line L1563 (28.342, 23.941) -> (29.342, 23.941)
  line L1564 (26.792, 32.434) -> (26.792, 31.434)
  line L1565 (26.792, 31.434) -> (27.792, 31.434)
  line L1566 (27.792, 31.434) -> (27.792, 32.434)
  line L1567 (27.792, 32.434) -> (26.792, 32.434)
  line L1568 (26.792, 31.634) -> (26.792, 30.634)
  line L1569 (26.792, 30.634) -> (27.792, 30.634)
  line L1570 (27.792, 30.634) -> (27.792, 31.634)
  line L1571 (27.792, 31.634) -> (26.792, 31.634)
  line L1572 (26.792, 30.834) -> (26.792, 29.834)
  line L1573 (26.792, 29.834) -> (27.792, 29.834)
  line L1574 (27.792, 29.834) -> (27.792, 30.834)
  line L1575 (27.792, 30.834) -> (26.792, 30.834)
  line L1576 (26.792, 30.034) -> (26.792, 29.034)
  line L1577 (26.792, 29.034) -> (27.792, 29.034)
  line L1578 (27.792, 29.034) -> (27.792, 30.034)
  line L1579 (27.792, 30.034) -> (26.792, 30.034)
  line L1580 (29.342, 29.034) -> (29.342, 30.034)
  line L1581 (29.342, 30.034) -> (28.342, 30.034)
  line L1582 (28.342, 30.034) -> (28.342, 29.034)
  line L1583 (28.342, 29.034) -> (29.342, 29.034)
  line L1584 (29.342, 29.834) -> (29.342, 30.834)
  line L1585 (29.342, 30.834) -> (28.342, 30.834)
  line L1586 (28.342, 30.834) -> (28.342, 29.834)
  line L1587 (28.342, 29.834) -> (29.342, 29.834)
  line L1588 (29.342, 30.634) -> (29.342, 31.634)
  line L1589 (29.342, 31.634) -> (28.342, 31.634)
  line L1590 (28.342, 31.634) -> (28.342, 30.634)
  line L1591 (28.342, 30.634) -> (29.342, 30.634)
  line L1592 (29.342, 31.434) -> (29.342, 32.434)
  line L1593 (29.342, 32.434) -> (28.342, 32.434)
  line L1594 (28.342, 32.434) -> (28.342, 31.434)
  line L1595 (28.342, 31.434) -> (29.342, 31.434)
  line L1596 (13.7, 30.325) -> (14.7, 30.325)
  line L1597 (14.7, 30.325) -> (14.7, 31.325)
  line L1598 (14.7, 31.325) -> (13.7, 31.325)
  line L1599 (13.7, 31.325) -> (13.7, 30.325)
  line L1600 (14.5, 30.325) -> (15.5, 30.325)
  line L1601 (15.5, 30.325) -> (15.5, 31.325)
  line L1602 (15.5, 31.325) -> (14.5, 31.325)
  line L1603 (14.5, 31.325) -> (14.5, 30.325)
  line L1604 (15.5, 32.875) -> (14.5, 32.875)
  line L1605 (14.5, 32.875) -> (14.5, 31.875)
  line L1606 (14.5, 31.875) -> (15.5, 31.875)
  line L1607 (15.5, 31.875) -> (15.5, 32.875)
  line L1608 (14.7, 32.875) -> (13.7, 32.875)
  line L1609 (13.7, 32.875) -> (13.7, 31.875)
  line L1610 (13.7, 31.875) -> (14.7, 31.875)
  line L1611 (14.7, 31.875) -> (14.7, 32.875)
  line L1612 (13.7367, 24.3158) -> (14.7367, 24.3158)
  line L1613 (14.7367, 24.3158) -> (14.7367, 25.3158)
  line L1614 (14.7367, 25.3158) -> (13.7367, 25.3158)
  line L1615 (13.7367, 25.3158) -> (13.7367, 24.3158)
  line L1616 (15.4512, 24.3158) -> (16.4512, 24.3158)
  line L1617 (16.4512, 24.3158) -> (16.4512, 25.3158)
  line L1618 (16.4512, 25.3158) -> (15.4512, 25.3158)
  line L1619 (15.4512, 25.3158) -> (15.4512, 24.3158)
  line L1620 (13.7367, 24.3412) -> (14.7367, 24.3412)
  line L1621 (14.7367, 24.3412) -> (14.7367, 25.3412)
  line L1622 (14.7367, 25.3412) -> (13.7367, 25.3412)
  line L1623 (13.7367, 25.3412) -> (13.7367, 24.3412)
  line L1624 (15.4512, 24.3412) -> (16.4512, 24.3412)
  line L1625 (16.4512, 24.3412) -> (16.4512, 25.3412)
  line L1626 (16.4512, 25.3412) -> (15.4512, 25.3412)
  line L1627 (15.4512, 25.3412) -> (15.4512, 24.3412)
  line L1628 (13.7748, 24.3666) -> (14.7748, 24.3666)
  line L1629 (14.7748, 24.3666) -> (14.7748, 25.3666)
  line L1630 (14.7748, 25.3666) -> (13.7748, 25.3666)
  line L1631 (13.7748, 25.3666) -> (13.7748, 24.3666)
  line L1632 (15.4512, 24.3666) -> (16.4512, 24.3666)
  line L1633 (16.4512, 24.3666) -> (16.4512, 25.3666)
  line L1634 (16.4512, 25.3666) -> (15.4512, 25.3666)
  line L1635 (15.4512, 25.3666) -> (15.4512, 24.3666)
  line L1636 (13.8256, 24.392) -> (14.8256, 24.392)
  line L1637 (14.8256, 24.392) -> (14.8256, 25.392)
  line L1638 (14.8256, 25.392) -> (13.8256, 25.392)
  line L1639 (13.8256, 25.392) -> (13.8256, 24.392)
  line L1640 (15.4512, 24.392) -> (16.4512, 24.392)
  line L1641 (16.4512, 24.392) -> (16.4512, 25.392)
  line L1642 (16.4512, 25.392) -> (15.4512, 25.392)
  line L1643 (15.4512, 25.392) -> (15.4512, 24.392)
  line L1644 (13.7287, 24.9047) -> (13.7541, 24.9047)
  line L1645 (13.7541, 24.9047) -> (13.7541, 24.9301)
  line L1646 (13.7541, 24.9301) -> (13.7287, 24.9301)
  line L1647 (13.7287, 24.9301) -> (13.7287, 24.9047)
  line L1648 (13.851, 24.4174) -> (14.851, 24.4174)
  line L1649 (14.851, 24.4174) -> (14.851, 25.4174)
  line L1650 (14.851, 25.4174) -> (13.851, 25.4174)
  line L1651 (13.851, 25.4174) -> (13.851, 24.4174)
  line L1652 (15.4512, 24.4174) -> (16.4512, 24.4174)
  line L1653 (16.4512, 24.4174) -> (16.4512, 25.4174)
  line L1654 (16.4512, 25.4174) -> (15.4512, 25.4174)
  line L1655 (15.4512, 25.4174) -> (15.4512, 24.4174)
  line L1656 (13.216, 24.4428) -> (14.216, 24.4428)
  line L1657 (14.216, 24.4428) -> (14.216, 25.4428)
  line L1658 (14.216, 25.4428) -> (13.216, 25.4428)
  line L1659 (13.216, 25.4428) -> (13.216, 24.4428)
  line L1660 (13.8764, 24.4428) -> (14.8764, 24.4428)
  line L1661 (14.8764, 24.4428) -> (14.8764, 25.4428)
  line L1662 (14.8764, 25.4428) -> (13.8764, 25.4428)
  line L1663 (13.8764, 25.4428) -> (13.8764, 24.4428)
  line L1664 (15.4512, 24.4428) -> (16.4512, 24.4428)
  line L1665 (16.4512, 24.4428) -> (16.4512, 25.4428)
  line L1666 (16.4512, 25.4428) -> (15.4512, 25.4428)
  line L1667 (15.4512, 25.4428) -> (15.4512, 24.4428)
  line L1668 (13.1906, 24.4682) -> (14.1906, 24.4682)
  line L1669 (14.1906, 24.4682) -> (14.1906, 25.4682)
  line L1670 (14.1906, 25.4682) -> (13.1906, 25.4682)
  line L1671 (13.1906, 25.4682) -> (13.1906, 24.4682)
  line L1672 (13.9018, 24.4682) -> (14.9018, 24.4682)
  line L1673 (14.9018, 24.4682) -> (14.9018, 25.4682)
  line L1674 (14.9018, 25.4682) -> (13.9018, 25.4682)
  line L1675 (13.9018, 25.4682) -> (13.9018, 24.4682)
  line L1676 (15.4639, 24.4682) -> (16.4639, 24.4682)
  line L1677 (16.4639, 24.4682) -> (16.4639, 25.4682)
  line L1678 (16.4639, 25.4682) -> (15.4639, 25.4682)
  line L1679 (15.4639, 25.4682) -> (15.4639, 24.4682)
  line L1680 (13.1652, 24.4936) -> (14.1652, 24.4936)
  line L1681 (14.1652, 24.4936) -> (14.1652, 25.4936)
  line L1682 (14.1652, 25.4936) -> (13.1652, 25.4936)
  line L1683 (13.1652, 25.4936) -> (13.1652, 24.4936)
  line L1684 (13.9272, 24.4936) -> (14.9272, 24.4936)
  line L1685 (14.9272, 24.4936) -> (14.9272, 25.4936)
  line L1686 (14.9272, 25.4936) -> (13.9272, 25.4936)
  line L1687 (13.9272, 25.4936) -> (13.9272, 24.4936)
  line L1688 (15.4639, 24.4936) -> (16.4639, 24.4936)
  line L1689 (16.4639, 24.4936) -> (16.4639, 25.4936)
  line L1690 (16.4639, 25.4936) -> (15.4639, 25.4936)
  line L1691 (15.4639, 25.4936) -> (15.4639, 24.4936)
  line L1692 (13.1525, 24.519) -> (14.1525, 24.519)
  line L1693 (14.1525, 24.519) -> (14.1525, 25.519)
  line L1694 (14.1525, 25.519) -> (13.1525, 25.519)
  line L1695 (13.1525, 25.519) -> (13.1525, 24.519)
  line L1696 (13.9526, 24.519) -> (14.9526, 24.519)
  line L1697 (14.9526, 24.519) -> (14.9526, 25.519)
  line L1698 (14.9526, 25.519) -> (13.9526, 25.519)
  line L1699 (13.9526, 25.519) -> (13.9526, 24.519)
  line L1700 (15.4639, 24.519) -> (16.4639, 24.519)
  line L1701 (16.4639, 24.519) -> (16.4639, 25.519)
  line L1702 (16.4639, 25.519) -> (15.4639, 25.519)
  line L1703 (15.4639, 25.519) -> (15.4639, 24.519)
  line L1704 (13.1271, 24.5444) -> (14.1271, 24.5444)
  line L1705 (14.1271, 24.5444) -> (14.1271, 25.5444)
  line L1706 (14.1271, 25.5444) -> (13.1271, 25.5444)
  line L1707 (13.1271, 25.5444) -> (13.1271, 24.5444)
  line L1708 (13.9653, 24.5444) -> (14.9653, 24.5444)
  line L1709 (14.9653, 24.5444) -> (14.9653, 25.5444)
  line L1710 (14.9653, 25.5444) -> (13.9653, 25.5444)
  line L1711 (13.9653, 25.5444) -> (13.9653, 24.5444)
  line L1712 (15.4639, 24.5444) -> (16.4639, 24.5444)
  line L1713 (16.4639, 24.5444) -> (16.4639, 25.5444)
  line L1714 (16.4639, 25.5444) -> (15.4639, 25.5444)
  line L1715 (15.4639, 25.5444) -> (15.4639, 24.5444)
  line L1716 (13.1144, 24.5698) -> (14.1144, 24.5698)
  line L1717 (14.1144, 24.5698) -> (14.1144, 25.5698)
  line L1718 (14.1144, 25.5698) -> (13.1144, 25.5698)
  line L1719 (13.1144, 25.5698) -> (13.1144, 24.5698)
  line L1720 (13.9907, 24.5698) -> (14.9907, 24.5698)
  line L1721 (14.9907, 24.5698) -> (14.9907, 25.5698)
  line L1722 (14.9907, 25.5698) -> (13.9907, 25.5698)
  line L1723 (13.9907, 25.5698) -> (13.9907, 24.5698)
  line L1724 (15.4639, 24.5698) -> (16.4639, 24.5698)
  line L1725 (16.4639, 24.5698) -> (16.4639, 25.5698)
  line L1726 (16.4639, 25.5698) -> (15.4639, 25.5698)
  line L1727 (15.4639, 25.5698) -> (15.4639, 24.5698)
  line L1728 (13.1017, 24.5952) -> (14.1017, 24.5952)
  line L1729 (14.1017, 24.5952) -> (14.1017, 25.5952)
  line L1730 (14.1017, 25.5952) -> (13.1017, 25.5952)
  line L1731 (13.1017, 25.5952) -> (13.1017, 24.5952)
  line L1732 (14.0034, 24.5952) -> (15.0034, 24.5952)
  line L1733 (15.0034, 24.5952) -> (15.0034, 25.5952)
  line L1734 (15.0034, 25.5952) -> (14.0034, 25.5952)
  line L1735 (14.0034, 25.5952) -> (14.0034, 24.5952)
  line L1736 (15.4639, 24.5952) -> (16.4639, 24.5952)
  line L1737 (16.4639, 24.5952) -> (16.4639, 25.5952)
  line L1738 (16.4639, 25.5952) -> (15.4639, 25.5952)
  line L1739 (15.4639, 25.5952) -> (15.4639, 24.5952)
  line L1740 (13.0763, 24.6206) -> (14.0763, 24.6206)
  line L1741 (14.0763, 24.6206) -> (14.0763, 25.6206)
  line L1742 (14.0763, 25.6206) -> (13.0763, 25.6206)
  line L1743 (13.0763, 25.6206) -> (13.0763, 24.6206)
  line L1744 (13.978, 24.6206) -> (14.978, 24.6206)
  line L1745 (14.978, 24.6206) -> (14.978, 25.6206)
  line L1746 (14.978, 25.6206) -> (13.978, 25.6206)
  line L1747 (13.978, 25.6206) -> (13.978, 24.6206)
  line L1748 (15.4639, 24.6206) -> (16.4639, 24.6206)
  line L1749 (16.4639, 24.6206) -> (16.4639, 25.6206)
  line L1750 (16.4639, 25.6206) -> (15.4639, 25.6206)
  line L1751 (15.4639, 25.6206) -> (15.4639, 24.6206)
  line L1752 (13.0636, 24.646) -> (14.0636, 24.646)
  line L1753 (14.0636, 24.646) -> (14.0636, 25.646)
  line L1754 (14.0636, 25.646) -> (13.0636, 25.646)
  line L1755 (13.0636, 25.646) -> (13.0636, 24.646)
  line L1756 (13.9526, 24.646) -> (14.9526, 24.646)
  line L1757 (14.9526, 24.646) -> (14.9526, 25.646)
  line L1758 (14.9526, 25.646) -> (13.9526, 25.646)
  line L1759 (13.9526, 25.646) -> (13.9526, 24.646)
  line L1760 (15.4639, 24.646) -> (16.4639, 24.646)
  line L1761 (16.4639, 24.646) -> (16.4639, 25.646)
  line L1762 (16.4639, 25.646) -> (15.4639, 25.646)
  line L1763 (15.4639, 25.646) -> (15.4639, 24.646)
  line L1764 (13.0509, 24.6714) -> (14.0509, 24.6714)
  line L1765 (14.0509, 24.6714) -> (14.0509, 25.6714)
  line L1766 (14.0509, 25.6714) -> (13.0509, 25.6714)
  line L1767 (13.0509, 25.6714) -> (13.0509, 24.6714)
  line L1768 (13.9272, 24.6714) -> (14.9272, 24.6714)
  line L1769 (14.9272, 24.6714) -> (14.9272, 25.6714)
  line L1770 (14.9272, 25.6714) -> (13.9272, 25.6714)
  line L1771 (13.9272, 25.6714) -> (13.9272, 24.6714)
  line L1772 (15.4766, 24.6714) -> (16.4766, 24.6714)
  line L1773 (16.4766, 24.6714) -> (16.4766, 25.6714)
  line L1774 (16.4766, 25.6714) -> (15.4766, 25.6714)
  line L1775 (15.4766, 25.6714) -> (15.4766, 24.6714)
  line L1776 (13.0382, 24.6968) -> (14.0382, 24.6968)
  line L1777 (14.0382, 24.6968) -> (14.0382, 25.6968)
  line L1778 (14.0382, 25.6968) -> (13.0382, 25.6968)
  line L1779 (13.0382, 25.6968) -> (13.0382, 24.6968)
  line L1780 (13.9145, 24.6968) -> (14.9145, 24.6968)
  line L1781 (14.9145, 24.6968) -> (14.9145, 25.6968)
  line L1782 (14.9145, 25.6968) -> (13.9145, 25.6968)
  line L1783 (13.9145, 25.6968) -> (13.9145, 24.6968)
  line L1784 (15.4766, 24.6968) -> (16.4766, 24.6968)
  line L1785 (16.4766, 24.6968) -> (16.4766, 25.6968)
  line L1786 (16.4766, 25.6968) -> (15.4766, 25.6968)
  line L1787 (15.4766, 25.6968) -> (15.4766, 24.6968)
  line L1788 (13.0255, 24.7222) -> (14.0255, 24.7222)
  line L1789 (14.0255, 24.7222) -> (14.0255, 25.7222)
  line L1790 (14.0255, 25.7222) -> (13.0255, 25.7222)
  line L1791 (13.0255, 25.7222) -> (13.0255, 24.7222)
  line L1792 (13.8891, 24.7222) -> (14.8891, 24.7222)
  line L1793 (14.8891, 24.7222) -> (14.8891, 25.7222)
  line L1794 (14.8891, 25.7222) -> (13.8891, 25.7222)
  line L1795 (13.8891, 25.7222) -> (13.8891, 24.7222)
  line L1796 (15.4766, 24.7222) -> (16.4766, 24.7222)
  line L1797 (16.4766, 24.7222) -> (16.4766, 25.7222)
  line L1798 (16.4766, 25.7222) -> (15.4766, 25.7222)
  line L1799 (15.4766, 25.7222) -> (15.4766, 24.7222)
  line L1800 (13.0128, 24.7476) -> (14.0128, 24.7476)
  line L1801 (14.0128, 24.7476) -> (14.0128, 25.7476)
  line L1802 (14.0128, 25.7476) -> (13.0128, 25.7476)
  line L1803 (13.0128, 25.7476) -> (13.0128, 24.7476)
  line L1804 (13.8637, 24.7476) -> (14.8637, 24.7476)
  line L1805 (14.8637, 24.7476) -> (14.8637, 25.7476)
  line L1806 (14.8637, 25.7476) -> (13.8637, 25.7476)
  line L1807 (13.8637, 25.7476) -> (13.8637, 24.7476)
  line L1808 (14.6892, 24.7476) -> (15.6892, 24.7476)
  line L1809 (15.6892, 24.7476) -> (15.6892, 25.7476)
  line L1810 (15.6892, 25.7476) -> (14.6892, 25.7476)
  line L1811 (14.6892, 25.7476) -> (14.6892, 24.7476)
  line L1812 (15.4766, 24.7476) -> (16.4766, 24.7476)
  line L1813 (16.4766, 24.7476) -> (16.4766, 25.7476)
  line L1814 (16.4766, 25.7476) -> (15.4766, 25.7476)
  line L1815 (15.4766, 25.7476) -> (15.4766, 24.7476)
  line L1816 (15.9973, 24.7476) -> (16.9973, 24.7476)
  line L1817 (16.9973, 24.7476) -> (16.9973, 25.7476)
  line L1818 (16.9973, 25.7476) -> (15.9973, 25.7476)
  line L1819 (15.9973, 25.7476) -> (15.9973, 24.7476)
  line L1820 (17.1403, 24.7476) -> (18.1403, 24.7476)
  line L1821 (18.1403, 24.7476) -> (18.1403, 25.7476)
  line L1822 (18.1403, 25.7476) -> (17.1403, 25.7476)
  line L1823 (17.1403, 25.7476) -> (17.1403, 24.7476)
  line L1824 (13.0001, 24.773) -> (14.0001, 24.773)
  line L1825 (14.0001, 24.773) -> (14.0001, 25.773)
  line L1826 (14.0001, 25.773) -> (13.0001, 25.773)
  line L1827 (13.0001, 25.773) -> (13.0001, 24.773)
  line L1828 (13.8383, 24.773) -> (14.8383, 24.773)
  line L1829 (14.8383, 24.773) -> (14.8383, 25.773)
  line L1830 (14.8383, 25.773) -> (13.8383, 25.773)
  line L1831 (13.8383, 25.773) -> (13.8383, 24.773)
  line L1832 (14.6765, 24.773) -> (15.6765, 24.773)
  line L1833 (15.6765, 24.773) -> (15.6765, 25.773)
  line L1834 (15.6765, 25.773) -> (14.6765, 25.773)
  line L1835 (14.6765, 25.773) -> (14.6765, 24.773)
  line L1836 (15.4766, 24.773) -> (16.4766, 24.773)
  line L1837 (16.4766, 24.773) -> (16.4766, 25.773)
  line L1838 (16.4766, 25.773) -> (15.4766, 25.773)
  line L1839 (15.4766, 25.773) -> (15.4766, 24.773)
  line L1840 (15.9973, 24.773) -> (16.9973, 24.773)
  line L1841 (16.9973, 24.773) -> (16.9973, 25.773)
  line L1842 (16.9973, 25.773) -> (15.9973, 25.773)
  line L1843 (15.9973, 25.773) -> (15.9973, 24.773)
  line L1844 (17.153, 24.773) -> (18.153, 24.773)
  line L1845 (18.153, 24.773) -> (18.153, 25.773)
  line L1846 (18.153, 25.773) -> (17.153, 25.773)
  line L1847 (17.153, 25.773) -> (17.153, 24.773)
  line L1848 (17.915, 24.773) -> (18.915, 24.773)
  line L1849 (18.915, 24.773) -> (18.915, 25.773)
  line L1850 (18.915, 25.773) -> (17.915, 25.773)
  line L1851 (17.915, 25.773) -> (17.915, 24.773)
  line L1852 (18.677, 24.773) -> (19.677, 24.773)
  line L1853 (19.677, 24.773) -> (19.677, 25.773)
  line L1854 (19.677, 25.773) -> (18.677, 25.773)
  line L1855 (18.677, 25.773) -> (18.677, 24.773)
  line L1856 (19.2358, 24.773) -> (20.2358, 24.773)
  line L1857 (20.2358, 24.773) -> (20.2358, 25.773)
  line L1858 (20.2358, 25.773) -> (19.2358, 25.773)
  line L1859 (19.2358, 25.773) -> (19.2358, 24.773)
  line L1860 (19.8327, 24.773) -> (20.8327, 24.773)
  line L1861 (20.8327, 24.773) -> (20.8327, 25.773)
  line L1862 (20.8327, 25.773) -> (19.8327, 25.773)
  line L1863 (19.8327, 25.773) -> (19.8327, 24.773)
  line L1864 (20.4677, 24.773) -> (21.4677, 24.773)
  line L1865 (21.4677, 24.773) -> (21.4677, 25.773)
  line L1866 (21.4677, 25.773) -> (20.4677, 25.773)
  line L1867 (20.4677, 25.773) -> (20.4677, 24.773)
  line L1868 (21.471, 24.773) -> (22.471, 24.773)
  line L1869 (22.471, 24.773) -> (22.471, 25.773)
  line L1870 (22.471, 25.773) -> (21.471, 25.773)
  line L1871 (21.471, 25.773) -> (21.471, 24.773)
  line L1872 (12.9874, 24.7984) -> (13.9874, 24.7984)
  line L1873 (13.9874, 24.7984) -> (13.9874, 25.7984)
  line L1874 (13.9874, 25.7984) -> (12.9874, 25.7984)
  line L1875 (12.9874, 25.7984) -> (12.9874, 24.7984)
  line L1876 (13.8256, 24.7984) -> (14.8256, 24.7984)
  line L1877 (14.8256, 24.7984) -> (14.8256, 25.7984)
  line L1878 (14.8256, 25.7984) -> (13.8256, 25.7984)
  line L1879 (13.8256, 25.7984) -> (13.8256, 24.7984)
  line L1880 (14.6765, 24.7984) -> (15.6765, 24.7984)
  line L1881 (15.6765, 24.7984) -> (15.6765, 25.7984)
  line L1882 (15.6765, 25.7984) -> (14.6765, 25.7984)
  line L1883 (14.6765, 25.7984) -> (14.6765, 24.7984)
  line L1884 (15.4766, 24.7984) -> (16.4766, 24.7984)
  line L1885 (16.4766, 24.7984) -> (16.4766, 25.7984)
  line L1886 (16.4766, 25.7984) -> (15.4766, 25.7984)
  line L1887 (15.4766, 25.7984) -> (15.4766, 24.7984)
  line L1888 (15.9846, 24.7984) -> (16.9846, 24.7984)
  line L1889 (16.9846, 24.7984) -> (16.9846, 25.7984)
  line L1890 (16.9846, 25.7984) -> (15.9846, 25.7984)
  line L1891 (15.9846, 25.7984) -> (15.9846, 24.7984)
  line L1892 (17.1276, 24.7984) -> (18.1276, 24.7984)
  line L1893 (18.1276, 24.7984) -> (18.1276, 25.7984)
  line L1894 (18.1276, 25.7984) -> (17.1276, 25.7984)
  line L1895 (17.1276, 25.7984) -> (17.1276, 24.7984)
  line L1896 (17.915, 24.7984) -> (18.915, 24.7984)
  line L1897 (18.915, 24.7984) -> (18.915, 25.7984)
  line L1898 (18.915, 25.7984) -> (17.915, 25.7984)
  line L1899 (17.915, 25.7984) -> (17.915, 24.7984)
  line L1900 (18.677, 24.7984) -> (19.677, 24.7984)
  line L1901 (19.677, 24.7984) -> (19.677, 25.7984)
  line L1902 (19.677, 25.7984) -> (18.677, 25.7984)
  line L1903 (18.677, 25.7984) -> (18.677, 24.7984)
  line L1904 (19.2358, 24.7984) -> (20.2358, 24.7984)
  line L1905 (20.2358, 24.7984) -> (20.2358, 25.7984)
  line L1906 (20.2358, 25.7984) -> (19.2358, 25.7984)
  line L1907 (19.2358, 25.7984) -> (19.2358, 24.7984)
  line L1908 (19.8454, 24.7984) -> (20.8454, 24.7984)
  line L1909 (20.8454, 24.7984) -> (20.8454, 25.7984)
  line L1910 (20.8454, 25.7984) -> (19.8454, 25.7984)
  line L1911 (19.8454, 25.7984) -> (19.8454, 24.7984)
  line L1912 (20.4677, 24.7984) -> (21.4677, 24.7984)